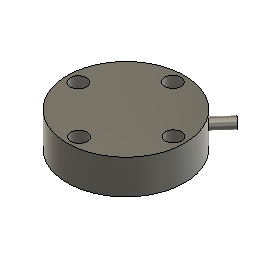
Final Assembly v4 (Autodesk Fusion 360 archive; units mm, degrees)
design "Compression Load Cell"
Autodesk Fusion 360 part; units mm, degrees
cylinder "CylinderPrimitive1" add diameter 29 height 8.5 placed x (1, 0, 0) y (0, 0, -1) z (0, 1, 0) at (0, 0, 0)
hole "Hole1" at (14.5, 3.75, 0) direction (-1, 0, 0) diameter 2.5 depth 0.5 tip angle 180
sketch "Sketch2" plane through (14, 0, 0) normal (1, 0, 0) x (0, 0, -1)
  circle A0 centre (0, 3.75) radius 1.25
  circle A1 centre (0, 3.75) radius 1.25
extrude "Extrude1" add sketch "Sketch2" along normal blind 5.5
move_body "Move1" bodies 1 to x (0.655619, 0, -0.755092) y (0, -1, 0) z (-0.755092, 0, -0.655619) at (0, 17, 0)
sketch "Sketch3" plane through (0, 17, 0) normal (0, 1, 0) x (-1, 0, 0)
  circle A0 centre (0, 0) radius 14.5
  circle A1 centre (-11.6825, -0.0908) radius 2
  dimension "d9" = 4
  measures "d9" diameter of A1
extrude "Extrude2" cut sketch "Sketch3" against normal blind 8.5 contours A1
pattern_circular "C-Pattern1" count 4 over 360 about axis through (0, 17, 0) along (0, 1, 0) of "Extrude2"
equation "d7 = 0.5 mm + 5 mm"

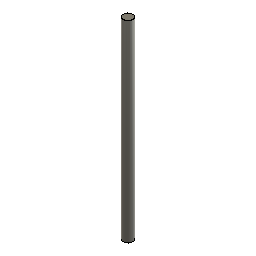
design "Locking Rod"
Autodesk Fusion 360 part; units mm, degrees
cylinder "CylinderPrimitive1" add diameter 4.95 height 100 placed x (1, 0, 0) y (0, 0, -1) z (0, 1, 0) at (0, 0, 0)
fillet "Fillet1" radius 0.1 2 edges at (-2.3075, 100, 0.895) (-2.3075, 0, -0.895)

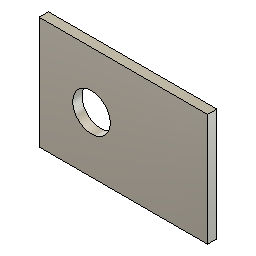
design "Left_Joint_Revolute"
Autodesk Fusion 360 part; units mm, degrees
box "BoxPrimitive1" add length 60 width 90 height 5 placed x (0, 1, 0) y (-1, 0, 0) z (0, 0, 1) at (55, -25, 0)
sketch "Sketch2" plane through (0, 0, 5) normal (0, 0, 1) x (1, 0, 0)
  line L0 (55, 35) -> (-35, 35)
  line L1 (-35, 35) -> (-35, -25)
  line L2 (-35, -25) -> (55, -25)
  line L3 (55, -25) -> (55, 35)
  circle A0 centre (-7, 5) radius 10.01
  dimension "d7" = 20.02
  measures "d7" diameter of A0
extrude "Extrude1" cut sketch "Sketch2" against normal blind 5 contours A0
equation "d7 = ( 10.01 * 2 ) * 1 mm"

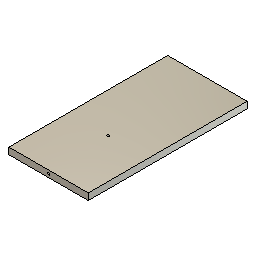
design "Right Joint Base"
Autodesk Fusion 360 part; units mm, degrees
box "BoxPrimitive1" add length 120 width 60 height 5 placed x (0, 0, -1) y (-1, 0, 0) z (0, 1, 0) at (45, 0, 20)
sketch "Sketch2" plane through (0, 0, -100) normal (0, 0, -1) x (-1, 0, 0)
  line L0 (-45, 5) -> (-45, 0)
  line L1 (-45, 0) -> (15, 0)
  line L2 (15, 0) -> (15, 5)
  line L3 (15, 5) -> (-45, 5)
  circle A0 centre (-15, 2.5) radius 0.8
  dimension "d6" = 1.6
  dimension "d6" = 1.6
  measures "d6" diameter of A0
extrude "Extrude1" cut sketch "Sketch2" against normal blind 20 contours A0
sketch "Sketch3" plane through (0, 0, 20) normal (0, 0, 1) x (1, 0, 0)
  line L0 (-15, 5) -> (-15, 0)
  line L1 (-15, 0) -> (45, 0)
  line L2 (45, 0) -> (45, 5)
  line L3 (45, 5) -> (-15, 5)
  circle A0 centre (15, 2.5) radius 0.8
  point P0 (15.8, 2.5)
  constraint coincident A0 P0
extrude "Extrude2" cut sketch "Sketch3" against normal blind 20 contours A0
sketch "Sketch4" plane through (0, 0, 0) normal (0, -1, 0) x (1, 0, 0)
  line L0 (-15, -100) -> (45, -100)
  line L1 (45, -100) -> (45, 20)
  line L2 (45, 20) -> (-15, 20)
  line L3 (-15, 20) -> (-15, -100)
  circle A0 centre (15, -25) radius 0.8
  point P0 (15.8, -100)
  dimension "d11" = 1.6
  measures "d11" diameter of A0
extrude "Extrude3" cut sketch "Sketch4" against normal blind 5 contours A0

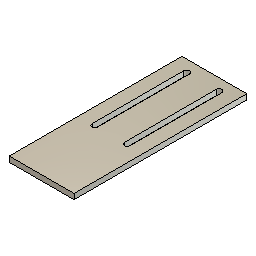
design "Extender_Left"
Autodesk Fusion 360 part; units mm, degrees
sketch "Sketch1" plane through (0, 0, 0) normal (0, 1, 0) x (1, 0, 0)
  line L0 (-20, 20) -> (40, 20)
  line L1 (40, 20) -> (40, -140)
  line L2 (40, -140) -> (-20, -140)
  line L3 (-20, -140) -> (-20, 20)
  dimension "d1" = 60
  dimension "d2" = 160
extrude "Extrude1" add sketch "Sketch1" along normal blind 5
sketch "Sketch2" plane through (0, 5, 0) normal (0, 1, 0) x (-1, 0, 0)
  circle A0 centre (-25, -9.2974) radius 2.625
  circle A1 centre (-25, 75.7026) radius 2.625
  line L0 (-27.625, -9.2836) -> (-27.625, 75.7026)
  line L1 (-22.3751, -9.3188) -> (-22.375, 75.7026)
  line L2 (-25, 75.7026) -> (5, 75.7026)
  circle A2 centre (5, 75.7026) radius 2.625
  line L3 (-25, -9.2974) -> (5, -9.2974)
  circle A3 centre (5, -9.2974) radius 2.625
  line L4 (2.375, -9.2974) -> (2.375, 75.7026)
  line L5 (7.625, 75.7026) -> (7.625, -9.2974)
  line L6 (-40, -20) -> (20, -20)
  line L7 (20, -20) -> (20, 140)
  dimension "d27" = 5.25
  dimension "d29" = 85
  dimension "d30" = 5.25
  dimension "d36" = 30
  dimension "d37" = 5.25
  dimension "d38" = 30
  dimension "d39" = 5.25
  measures "d27" diameter of A0
  measures "d29" distance of origin
  measures "d30" diameter of A1
  measures "d36" distance of origin
  measures "d37" diameter of A2
  measures "d39" diameter of A3
extrude "Extrude2" cut sketch "Sketch2" against normal blind 5 contours A0 | A0 A1 L0 L1 | A1 | A2 A3 L4 L5 | A3 | A2

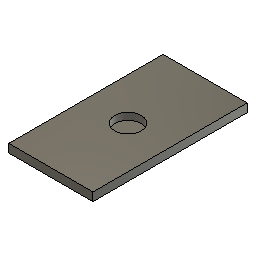
design "U Plate"
Autodesk Fusion 360 part; units mm, degrees
box "BoxPrimitive1" add length 110 width 60 height 6 placed x (0, 0, 1) y (1, 0, 0) z (0, 1, 0) at (0, 0, 0)
sketch "Sketch3" plane through (0, 6, 0) normal (0, 1, 0) x (-1, 0, 0)
  line L0 (0, 110) -> (-60, 110)
  line L1 (-60, 110) -> (-60, 0)
  line L2 (-60, 0) -> (0, 0)
  line L3 (0, 0) -> (0, 110)
  circle A0 centre (-30, 55) radius 9.5
  dimension "d6" = 19
  measures "d6" diameter of A0
extrude "Extrude1" cut sketch "Sketch3" against normal blind 5 contours A0
equation "d6 = ( 9.5 * 2 ) * 1 mm"

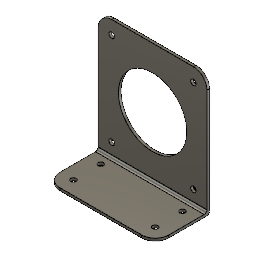
design "L-Clamp"
Autodesk Fusion 360 part; units mm, degrees
sketch "Sketch1" plane through (0, 0, 0) normal (0, 1, 0) x (1, 0, 0)
  line L0 (10, -10) -> (50, -10)
  line L1 (50, -10) -> (50, -30)
  line L2 (50, -30) -> (10, -30)
  line L3 (10, -30) -> (10, -10)
  line L4 (10, -10) -> (15, -10)
  circle A0 centre (15, -15) radius 1
  circle A1 centre (15, -25) radius 1
  circle A2 centre (45, -15) radius 1
  circle A3 centre (45, -25) radius 1
  dimension "d1" = 40
  dimension "d2" = 20
  dimension "d3" = 5
  dimension "d5" = 2
  dimension "d7" = 2
  dimension "d9" = 2
  dimension "d10" = 2
  measures "d5" diameter of A0
  measures "d7" diameter of A1
  measures "d9" diameter of A2
  measures "d10" diameter of A3
extrude "Extrude1" add sketch "Sketch1" along normal blind 1
sketch "Sketch2" plane through (0, 1, 0) normal (0, 1, 0) x (-1, 0, 0)
  circle A0 centre (-15, 25) radius 1
  circle A1 centre (-45, 15) radius 1
  circle A2 centre (-45, 25) radius 1
  circle A3 centre (-15, 15) radius 1
  line L0 (-10, 10) -> (-10, 30)
  line L1 (-10, 30) -> (-50, 30)
  line L2 (-50, 30) -> (-50, 10)
  line L3 (-50, 10) -> (-10, 10)
  line L4 (-10, 10) -> (-50, 10)
  line L5 (-50, 10) -> (-50, 11)
  line L6 (-50, 11) -> (-10, 11)
  line L7 (-10, 11) -> (-10, 10)
extrude "Extrude2" add sketch "Sketch2" along normal blind 44 contours L0 L2 L3 L4 L5 L6 L7
sketch "Sketch3" plane through (0, 0, 11) normal (0, 0, 1) x (1, 0, 0)
  line L0 (10, 1) -> (50, 1)
  line L1 (50, 1) -> (50, 45)
  line L2 (50, 45) -> (10, 45)
  line L3 (10, 45) -> (10, 1)
  circle A0 centre (30, 23) radius 12.5
  circle A1 centre (15, 6) radius 1
  circle A2 centre (45, 6) radius 1
  circle A3 centre (15, 40) radius 1
  circle A4 centre (45, 40) radius 1
  dimension "d15" = 25
  dimension "d17" = 2
  dimension "d19" = 2
  dimension "d21" = 2
  dimension "d22" = 2
  measures "d15" diameter of A0
  measures "d17" diameter of A1
  measures "d19" diameter of A2
  measures "d21" diameter of A3
  measures "d22" diameter of A4
extrude "Extrude3" cut sketch "Sketch3" against normal blind 1 contours A0 | A1 | A2 | A3 | A4
fillet "Fillet1" radius 5 4 edges at (50, 45, 10.5) (10, 45, 10.5) (50, 0.5, 30) (10, 0.5, 30)
fillet "Fillet2" radius 1 2 edges at (30, 0, 10) (30, 1, 11)

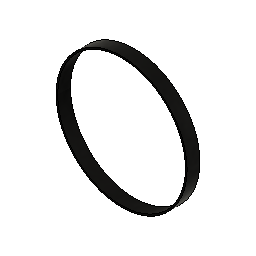
design "Wheel Rubber"
Autodesk Fusion 360 part; units mm, degrees
sketch "Sketch1" plane through (0, 0, 0) normal (0, 0, 1) x (1, 0, 0)
  circle A0 centre (0, 0) radius 10.25
  circle A1 centre (0, 0) radius 10
  dimension "d1" = 20.5
  dimension "d2" = 20
  measures "d1" diameter of A0
  measures "d2" diameter of A1
extrude "Extrude1" add sketch "Sketch1" along normal blind 2

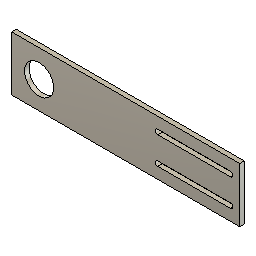
design "Right Joint Non-gear Side"
Autodesk Fusion 360 part; units mm, degrees
box "BoxPrimitive1" add length 60 width 250 height 5 placed x (0, 1, 0) y (-1, 0, 0) z (0, 0, 1) at (205, -35, 0)
sketch "Sketch2" plane through (0, 0, 0) normal (0, 0, -1) x (-1, 0, 0)
  line L0 (45, 25) -> (-205, 25)
  line L1 (-205, 25) -> (-205, -35)
  line L2 (-205, -35) -> (45, -35)
  line L3 (45, -35) -> (45, 25)
  circle A0 centre (15, -5) radius 15.984
  circle A1 centre (-195, -20) radius 2.625
  circle A2 centre (-195, 10) radius 2.625
  line L4 (-195, 12.625) -> (-115, 12.625)
  line L5 (-195, 7.375) -> (-115, 7.375)
  circle A3 centre (-115, 10) radius 2.625
  line L6 (-195, -17.375) -> (-115, -17.375)
  line L7 (-195, -22.625) -> (-115, -22.625)
  circle A4 centre (-115, -20) radius 2.625
  dimension "d9" = 31.968
  dimension "d12" = 5.25
  dimension "d14" = 5.25
  dimension "d15" = 80
  dimension "d16" = 80
  dimension "d17" = 80
  dimension "d18" = 80
  measures "d9" diameter of A0
  measures "d12" diameter of A1
  measures "d14" diameter of A2
extrude "Extrude1" cut sketch "Sketch2" against normal blind 5 contours A0 | A1 | A1 L6 L7 A4 | A4 | A2 | A2 L4 L5 A3 | A3

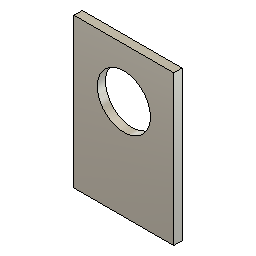
design "Right Joint Revolute Part"
Autodesk Fusion 360 part; units mm, degrees
box "BoxPrimitive1" add length 90 width 60 height 5 placed x (0, 1, 0) y (-1, 0, 0) z (0, 0, 1) at (50, 30, 0)
sketch "Sketch3" plane through (0, 0, 5) normal (0, 0, 1) x (1, 0, 0)
  line L0 (50, 120) -> (-10, 120)
  line L1 (-10, 120) -> (-10, 30)
  line L2 (-10, 30) -> (50, 30)
  line L3 (50, 30) -> (50, 120)
  circle A0 centre (20, 90) radius 15.984
  dimension "d7" = 31.968
  measures "d7" diameter of A0
extrude "Extrude1" cut sketch "Sketch3" against normal blind 5 contours A0
sketch "Sketch4" plane through (0, 30, 0) normal (0, -1, 0) x (1, 0, 0)
  line L0 (-10, 5) -> (-10, 0)
  line L1 (-10, 0) -> (50, 0)
  line L2 (50, 0) -> (50, 5)
  line L3 (50, 5) -> (-10, 5)
  circle A0 centre (20, 2.5) radius 0.8
  dimension "d10" = 1.6
  measures "d10" diameter of A0
extrude "Extrude2" cut sketch "Sketch4" against normal blind 20 contours A0

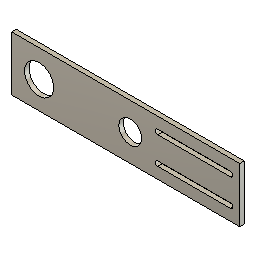
design "Right Joint Gear Side"
Autodesk Fusion 360 part; units mm, degrees
box "BoxPrimitive1" add length 60 width 250 height 5 placed x (0, 1, 0) y (-1, 0, 0) z (0, 0, 1) at (205, -35, 0)
sketch "Sketch2" plane through (0, 0, 0) normal (0, 0, -1) x (-1, 0, 0)
  line L0 (45, 25) -> (-205, 25)
  line L1 (-205, 25) -> (-205, -35)
  line L2 (-205, -35) -> (45, -35)
  line L3 (45, -35) -> (45, 25)
  circle A0 centre (-85, -5) radius 12.5
  circle A1 centre (15, -5) radius 15.984
  dimension "d8" = 25
  dimension "d9" = 31.968
  measures "d8" diameter of A0
  measures "d9" diameter of A1
sketch "Sketch4" plane through (0, 0, 5) normal (0, 0, 1) x (1, 0, 0)
  line L0 (205, 25) -> (-45, 25)
  line L1 (-45, 25) -> (-45, -35)
  line L2 (-45, -35) -> (205, -35)
  line L3 (205, -35) -> (205, 25)
  circle A0 centre (195, -20) radius 2.625
  circle A1 centre (195, 10) radius 2.625
  line L4 (195, -22.625) -> (115, -22.625)
  line L5 (195, -17.375) -> (115, -17.375)
  circle A2 centre (115, -20) radius 2.625
  line L6 (195, 7.375) -> (115, 7.375)
  line L7 (195, 12.625) -> (115, 12.625)
  circle A3 centre (115, 10) radius 2.625
  dimension "d15" = 5.25
  dimension "d16" = 5.25
  dimension "d17" = 80
  dimension "d18" = 80
  dimension "d19" = 80
  dimension "d20" = 80
  measures "d15" diameter of A0
  measures "d16" diameter of A1
extrude "Extrude1" cut sketch "Sketch2" against normal blind 5 contours A0 | A1
extrude "Extrude2" cut sketch "Sketch4" against normal blind 5 contours A0 | A0 L4 L5 A2 | A2 | A1 | A1 L6 L7 A3 | A3

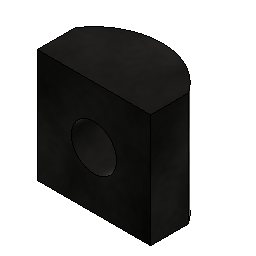
design "Rubber Stopper"
Autodesk Fusion 360 part; units mm, degrees
sketch "Sketch1" plane through (0, 0, 0) normal (0, 1, 0) x (1, 0, 0)
  line L0 (5, -10) -> (20, -10)
  line L1 (5, -10) -> (5, -5)
  line L2 (20, -10) -> (20, -5)
  arc A0 (20, -5) -> (5, -5) centre (12.5, -10) ccw
  dimension "d1" = 15
  dimension "d2" = 5
extrude "Extrude1" add sketch "Sketch1" along normal blind 15
sketch "Sketch2" plane through (0, 0, 10) normal (0, 0, 1) x (1, 0, 0)
  line L0 (5, 0) -> (20, 0)
  line L1 (20, 0) -> (20, 15)
  line L2 (20, 15) -> (5, 15)
  line L3 (5, 15) -> (5, 0)
  circle A0 centre (12.5, 7.5) radius 3
  dimension "d5" = 6
  measures "d5" diameter of A0
extrude "Extrude2" cut sketch "Sketch2" against normal blind 10 contours A0

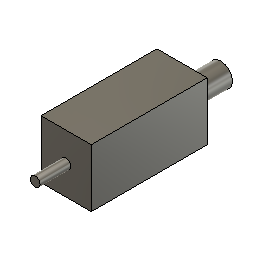
design "Solenoid"
Autodesk Fusion 360 part; units mm, degrees
box "BoxPrimitive1" add length 30 width 13 height 15 placed x (0, 0, -1) y (-1, 0, 0) z (0, 1, 0) at (13, 0, 30)
sketch "Sketch2" plane through (0, 0, 0) normal (0, 0, -1) x (-1, 0, 0)
  line L0 (-13, 15) -> (-13, 0)
  line L1 (-13, 0) -> (0, 0)
  line L2 (0, 0) -> (0, 15)
  line L3 (0, 15) -> (-13, 15)
  circle A0 centre (-6.5, 7.5) radius 3
  dimension "d6" = 6
  measures "d6" diameter of A0
extrude "Extrude1" add sketch "Sketch2" along normal blind 10 contours A0
sketch "Sketch3" plane through (0, 0, 30) normal (0, 0, 1) x (1, 0, 0)
  line L0 (0, 15) -> (0, 0)
  line L1 (0, 0) -> (13, 0)
  line L2 (13, 0) -> (13, 15)
  line L3 (13, 15) -> (0, 15)
  circle A0 centre (6.5, 7.5) radius 1.25
  dimension "d9" = 2.5
  measures "d9" diameter of A0
extrude "Extrude2" add sketch "Sketch3" along normal blind 8 contours A0

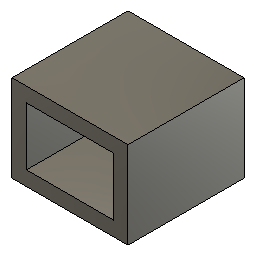
design "Fixture"
Autodesk Fusion 360 part; units mm, degrees
sketch "Sketch1" plane through (0, 0, 0) normal (0, 0, 1) x (1, 0, 0)
  line L0 (0, 0) -> (40, 0)
  line L1 (40, 0) -> (40, 30)
  line L2 (40, 30) -> (0, 30)
  line L3 (5, 5) -> (35, 5)
  line L4 (35, 5) -> (35, 25)
  line L5 (35, 25) -> (5, 25)
  line L6 (5, 25) -> (5, 5)
  line L7 (0, 30) -> (0, 0)
  dimension "d3" = 20
  dimension "d4" = 30
  dimension "d7" = 40
  dimension "d8" = 5
  dimension "d9" = 5
  dimension "d10" = 5
  measures "d3" distance of L0.start
  measures "d4" distance of L0.start
  measures "d7" distance of L0.start
  measures "d8" distance of L0 L3
  measures "d9" distance of L1 L4
  measures "d10" distance of L6 L7
extrude "Extrude1" add sketch "Sketch1" along normal blind 40

design "Leg"
Autodesk Fusion 360 part; units mm, degrees
sketch "Sketch1" plane through (0, 0, 0) normal (0, 1, 0) x (1, 0, 0)
  line L0 (-20, 25) -> (40, 25)
  line L1 (40, 25) -> (40, -145)
  line L2 (40, -145) -> (-20, -145)
  line L3 (-20, -145) -> (-20, 25)
  dimension "d1" = 60
  dimension "d2" = 170
extrude "Extrude1" add sketch "Sketch1" along normal blind 5
sketch "Sketch2" plane through (0, 5, 0) normal (0, 1, 0) x (-1, 0, 0)
  circle A0 centre (5, -14.9) radius 2.625
  circle A1 centre (-25, -14.9) radius 2.625
  line L0 (20, 145) -> (-40, 145)
  line L1 (-40, 145) -> (-40, -25)
  line L2 (-40, -25) -> (20, -25)
  line L3 (20, -25) -> (20, 145)
  dimension "d38" = 30
extrude "Extrude2" cut sketch "Sketch2" against normal blind 5 contours A0 | A1
sketch "Sketch6" plane through (0, 5, 0) normal (0, 1, 0) x (-1, 0, 0)
  circle A0 centre (5, -14.9) radius 2.625
  circle A1 centre (-25, -14.9) radius 2.625
  line L0 (20, 145) -> (-40, 145)
  line L1 (-40, 145) -> (-40, -25)
  line L2 (-40, -25) -> (20, -25)
  circle A2 centre (-30, 135) radius 2.5
  circle A3 centre (10, 135) radius 2.5
  circle A4 centre (-10, 135) radius 2.5
  dimension "d53" = 5
  dimension "d54" = 5
  dimension "d55" = 5
  measures "d53" diameter of A2
  measures "d54" diameter of A3
  measures "d55" diameter of A4
extrude "Extrude5" cut sketch "Sketch6" against normal blind 5 contours A2 | A3 | A4
sketch "Sketch7" plane through (0, 5, 0) normal (0, 1, 0) x (-1, 0, 0)
  circle A0 centre (10, 135) radius 2.5
  circle A1 centre (-10, 135) radius 2.5
  circle A2 centre (-30, 135) radius 2.5
  circle A3 centre (5, -14.9) radius 2.625
  circle A4 centre (-25, -14.9) radius 2.625
  line L0 (20, 145) -> (-40, 145)
  line L1 (-40, 145) -> (-40, -25)
  line L2 (-40, -25) -> (20, -25)
  line L3 (20, -25) -> (20, 145)
  circle A5 centre (-10, 112.5) radius 1.25
  dimension "d58" = 22.5
  dimension "d59" = 2.5
  measures "d59" diameter of A5
extrude "Extrude6" cut sketch "Sketch7" against normal blind 5 contours A5
equation "d59 = ( 1.25 * 2 ) * 1 mm"

design "Wheel"
Autodesk Fusion 360 part; units mm, degrees
sketch "Sketch1" plane through (0, 0, 0) normal (0, 1, 0) x (1, 0, 0)
  circle A0 centre (0, 0) radius 10
  circle A1 centre (0, 0) radius 3.5
  dimension "d1" = 20
  dimension "d2" = 7
  measures "d1" diameter of A0
  measures "d2" diameter of A1
extrude "Extrude1" add sketch "Sketch1" along normal blind 3

design "Wheel Shaft"
Autodesk Fusion 360 part; units mm, degrees
cylinder "CylinderPrimitive1" add diameter 7 height 95 placed x (1, 0, 0) y (0, 0, -1) z (0, 1, 0) at (0, 0, 0)
sketch "Sketch3" plane through (0, 0, 0) normal (0, -1, 0) x (1, 0, 0)
  circle A0 centre (0, 0) radius 3.5
  circle A1 centre (0, 0) radius 3
  dimension "d3" = 6
  measures "d3" diameter of A1
extrude "Extrude1" cut sketch "Sketch3" against normal blind 95 contours A1

design "Left_Joint_Base_Plate"
Autodesk Fusion 360 part; units mm, degrees
box "BoxPrimitive1" add length 120 width 60 height 5 placed x (0, 0, -1) y (-1, 0, 0) z (0, 1, 0) at (50, 0, 30)
sketch "Sketch5" plane through (0, 5, 0) normal (0, 1, 0) x (-1, 0, 0)
  line L0 (-50, -90) -> (10, -90)
  line L1 (10, -90) -> (10, 30)
  line L2 (10, 30) -> (-50, 30)
  line L3 (-50, 30) -> (-50, -90)
  circle A0 centre (-20, -2.5) radius 2.475
  circle A1 centre (-20, -27.5) radius 2.475
  dimension "d17" = 4.95
  dimension "d19" = 4.95
  measures "d17" diameter of A0
  measures "d19" diameter of A1
extrude "Extrude2" cut sketch "Sketch5" against normal blind 5 contours A0 | A1

design "Delarin Rod"
Autodesk Fusion 360 part; units mm, degrees
cylinder "CylinderPrimitive1" add diameter 8.1 height 240 placed x (1, 0, 0) y (0, 0, -1) z (0, 1, 0) at (0, 0, 0)
